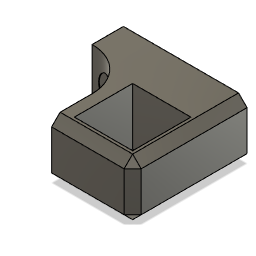
Hanger__Rod (Autodesk Fusion 360 design; units mm, degrees)
Autodesk Fusion 360 part; units mm, degrees
note: some values were not read from the file. Set by a fixed rule: which sketch regions a step uses.
sketch "Sketch1" plane through (0, 0, 0) normal (0, 1, 0) x (1, 0, 0)
  line L0 (0, 0) -> (20.5, 0)
  line L1 (20.5, 0) -> (20.5, -20.5)
  line L2 (20.5, -20.5) -> (0, -20.5)
  line L3 (0, -20.5) -> (0, 0)
  line L4 (0, 0) -> (-4, 0)
  line L5 (-4, 0) -> (-4, 4)
  line L6 (-4, 4) -> (0, 4)
  line L7 (0, 4) -> (0, 0)
  line L8 (-4, 4) -> (24.5, 4)
  line L9 (24.5, 4) -> (24.5, -24.5)
  line L10 (24.5, -24.5) -> (-4, -24.5)
  line L11 (-4, -24.5) -> (-4, 4)
  dimension "d1" = 20.5
  dimension "d2" = 20.5
  dimension "d3" = 4
  dimension "d4" = 4
  dimension "d5" = 28.5
  dimension "d6" = 28.5
  constraint horizontal L0
  constraint vertical L1
  constraint horizontal L2
  constraint vertical L3
  constraint coincident L0.start L3.end
  constraint horizontal L4
  constraint vertical L5
  constraint horizontal L6
  constraint vertical L7
  constraint horizontal L8
  constraint vertical L9
  constraint horizontal L10
  constraint vertical L11
  measures "d1" distance of L0.start L0.end
  measures "d2" distance of L0.start L2.end
  measures "d3" distance of L0.start L4.end
  measures "d4" distance of L0.start L6.end
  measures "d5" distance of L5.end L8.end
  measures "d6" distance of L5.end L10.end
extrude "Extrude1" add sketch "Sketch1" along normal blind 20
chamfer "Chamfer1" distance 3 angle 45 5 edges at (24.5, 20, 10.25) (10.25, 20, 24.5) (24.5, 10, 24.5) (24.5, 0, 10.25) (10.25, 0, 24.5)
sketch "Sketch2" plane through (0, 0, -4) normal (0, 0, -1) x (-1, 0, 0)
  line L0 (-24.5, 3) -> (-21.5, 0)
  line L1 (-21.5, 0) -> (4, 0)
  line L2 (4, 0) -> (4, 20)
  line L3 (4, 20) -> (-21.5, 20)
  line L4 (-21.5, 20) -> (-24.5, 17)
  line L5 (-24.5, 17) -> (-24.5, 3)
  line L6 (-24.5, 10) -> (-10.25, 10)
  line L7 (-7.6519, 5.5) -> (-5.0538, 10)
  line L8 (-5.0538, 10) -> (-7.6519, 14.5)
  line L9 (-7.6519, 14.5) -> (-12.8481, 14.5)
  line L10 (-12.8481, 14.5) -> (-15.4462, 10)
  line L11 (-15.4462, 10) -> (-12.8481, 5.5)
  line L12 (-12.8481, 5.5) -> (-7.6519, 5.5)
  point P0 (-10.25, 10)
  dimension "d10" = 14.25
  dimension "d11" = 4.5
  constraint midpoint L5 L6.start
  constraint perpendicular L2 L6
  constraint coincident P0 L6.end
  measures "d10" distance of L6.start P0
  measures "d11" distance of P0 L12
extrude "Extrude2" add sketch "Sketch2" along normal blind 4
sketch "Sketch3" plane through (0, 0, -8) normal (0, 0, -1) x (-1, 0, 0)
  line L0 (-7.6519, 5.5) -> (-12.8481, 5.5)
  line L1 (-15.4462, 10) -> (-12.8481, 14.5)
  line L2 (-12.8481, 14.5) -> (-7.6519, 14.5)
  line L3 (-7.6519, 14.5) -> (-5.0538, 10)
  line L4 (-5.0538, 10) -> (-7.6519, 5.5)
  line L5 (-24.5, 17) -> (-24.5, 3)
  line L6 (-24.5, 3) -> (-21.5, 0)
  line L7 (-21.5, 0) -> (4, 0)
  line L8 (4, 0) -> (4, 20)
  line L9 (4, 20) -> (-21.5, 20)
  line L10 (-21.5, 20) -> (-24.5, 17)
  line L11 (-7.6519, 14.5) -> (-5.0538, 14.5)
  line L12 (-5.0538, 14.5) -> (-5.0538, 10)
  line L13 (-15.4462, 10) -> (-15.4462, 14.5)
  line L14 (-15.4462, 14.5) -> (-12.8481, 14.5)
  constraint coincident L2.end L3.start
  constraint parallel L2 L11
  constraint coincident L3.end L4.start
  constraint perpendicular L11 L12
  constraint coincident L1.start L13.start
  constraint perpendicular L2 L13
  constraint coincident L1.end L2.start
  constraint perpendicular L13 L14
extrude "Extrude3" cut sketch "Sketch3" against normal blind 4 contours L1 L13 L14 | L3 L11 L12
sketch "Sketch4" plane through (0, 0, -8) normal (0, 0, -1) x (-1, 0, 0)
  line L0 (-15.4462, 14.5) -> (-5.0538, 14.5)
  line L1 (-5.0538, 14.5) -> (-5.0538, 10)
  line L2 (-5.0538, 10) -> (-7.6519, 5.5)
  line L3 (-7.6519, 5.5) -> (-12.8481, 5.5)
  line L4 (-12.8481, 5.5) -> (-15.4462, 10)
  line L5 (-15.4462, 10) -> (-15.4462, 14.5)
  line L6 (-24.5, 17) -> (-24.5, 3)
  line L7 (-24.5, 3) -> (-21.5, 0)
  line L8 (-21.5, 0) -> (4, 0)
  line L9 (4, 0) -> (4, 20)
  line L10 (4, 20) -> (-21.5, 20)
  line L11 (-21.5, 20) -> (-24.5, 17)
  line L12 (-10.25, 5.5) -> (-10.25, 10)
  circle A0 centre (-10.25, 10) radius 2
  line L13 (-5.0538, 14.5) -> (-15.4186, 14.5)
  line L14 (-15.4186, 14.5) -> (-15.4186, 5.5)
  line L15 (-15.4186, 5.5) -> (-5.0538, 5.5)
  line L16 (-5.0538, 5.5) -> (-5.0538, 14.5)
  line L17 (7, 22) -> (-27, 22)
  line L18 (-27, 22) -> (-27, -2)
  line L19 (-27, -2) -> (7, -2)
  line L20 (7, -2) -> (7, 22)
  dimension "d16" = 4
  constraint midpoint L3 L12.start
  constraint perpendicular L0 L12
  constraint coincident L12.end A0.centre
  constraint horizontal L13
  constraint vertical L14
  constraint horizontal L15
  constraint vertical L16
  constraint coincident L0.end L1.start
  constraint horizontal L17
  constraint vertical L18
  constraint horizontal L19
  constraint vertical L20
  measures "d16" diameter of A0
extrude "Extrude4" add sketch "Sketch4" along normal blind 5 contours L0 L1 L2 L3 L4 L13 L14 L15 L16 | L4 L14 L15 | L2 L15 L16 | L6 L7 L8 L9 L10 L11
extrude "Extrude5" add 1 faces at (0.0833, 10, -13) along direction (0, 0, -1) blind 1.75
sketch "Sketch5" plane through (-4, 0, 0) normal (-1, 0, 0) x (0, 0, 1)
  line L0 (21.5, 0) -> (24.5, 3)
  line L1 (24.5, 3) -> (24.5, 17)
  line L2 (24.5, 17) -> (21.5, 20)
  line L3 (21.5, 20) -> (-14.75, 20)
  line L4 (-14.75, 20) -> (-14.75, 0)
  line L5 (-14.75, 0) -> (21.5, 0)
  line L6 (-14.75, 20) -> (-4.75, 20)
  line L7 (-4.75, 20) -> (-4.75, 0)
  line L8 (-4.75, 0) -> (-14.75, 0)
  line L9 (-14.75, 0) -> (-14.75, 20)
  dimension "d21" = 10
  constraint horizontal L6
  constraint vertical L7
  constraint horizontal L8
  constraint vertical L9
  constraint coincident L3.end L4.start
  measures "d21" distance of L3.end L6.end
extrude "Extrude6" add sketch "Sketch5" along normal blind 15 contours L3 L4 L5 L6 L7 L8 L9
sketch "Sketch6" plane through (0, 0, -4.75) normal (0, 0, 1) x (1, 0, 0)
  line L0 (-4, 0) -> (-4, 20)
  line L1 (-4, 20) -> (-19, 20)
  line L2 (-19, 20) -> (-19, 0)
  line L3 (-19, 0) -> (-4, 0)
  line L4 (-19, 10) -> (-11.5, 10)
  circle A0 centre (-11.5, 10) radius 3.5
  dimension "d24" = 7.5
  dimension "d25" = 7
  constraint midpoint L2 L4.start
  constraint perpendicular L2 L4
  constraint coincident L4.end A0.centre
  measures "d24" distance of L4.start L4.end
  measures "d25" diameter of A0
extrude "Extrude7" cut sketch "Sketch6" against normal blind 10 contours A0
sketch "Sketch7" plane through (0, 0, 0) normal (0, -1, 0) x (1, 0, 0)
  line L0 (21.5, -14.75) -> (21.5, 21.5)
  line L1 (21.5, 21.5) -> (-4, 21.5)
  line L2 (-4, 21.5) -> (-4, -4.75)
  line L3 (-4, -4.75) -> (-19, -4.75)
  line L4 (-19, -4.75) -> (-19, -14.75)
  line L5 (-19, -14.75) -> (21.5, -14.75)
  line L6 (0, 20.5) -> (20.5, 20.5)
  line L7 (20.5, 20.5) -> (20.5, 0)
  line L8 (20.5, 0) -> (0, 0)
  line L9 (0, 0) -> (0, 20.5)
  line L10 (-19, -4.75) -> (-19, 10.25)
  circle A0 centre (-19, 10.25) radius 15
  dimension "d28" = 15
  constraint coincident L3.end L4.start
  constraint perpendicular L3 L10
  constraint coincident L10.end A0.centre
  constraint coincident L3.end A0
  measures "d28" distance of L3.end L10.end
extrude "Extrude8" add sketch "Sketch7" against normal blind 20 contours L2 L3 A0
sketch "Sketch8" plane through (0, 0, -14.75) normal (0, 0, -1) x (-1, 0, 0)
  circle A0 centre (11.5, 10) radius 3.5
  line L0 (-15.4462, 14.5) -> (-15.4186, 14.5)
  line L1 (-15.4186, 14.5) -> (-15.4186, 9.9523)
  line L2 (-15.4186, 9.9523) -> (-15.4462, 10)
  line L3 (-15.4462, 10) -> (-15.4462, 14.5)
  circle A1 centre (-10.25, 10) radius 2
  line L4 (-21.5, 20) -> (-24.5, 17)
  line L5 (-24.5, 17) -> (-24.5, 3)
  line L6 (-24.5, 3) -> (-21.5, 0)
  line L7 (-21.5, 0) -> (19, 0)
  line L8 (19, 0) -> (19, 20)
  line L9 (19, 20) -> (-21.5, 20)
  circle A2 centre (11.5, 10) radius 5
  dimension "d31" = 10
  constraint concentric A0 A2
  measures "d31" diameter of A2
extrude "Extrude9" cut sketch "Sketch8" along normal blind -10 and the other way blind 27 contours A2
extrude "Extrude10" cut 1 faces at (-11.9678, 9.7747, -4.75) along direction (0, 0, 1) blind 20
sketch "Sketch9" plane through (0, 0, -4.75) normal (0, 0, 1) x (1, 0, 0)
  circle A0 centre (-11.5, 10) radius 3.5
  circle A1 centre (-11.5, 10) radius 5
  circle A2 centre (-11.5, 10) radius 2
  dimension "d38" = 4
  constraint concentric A0 A2
  measures "d38" diameter of A2
extrude "Extrude11" add sketch "Sketch9" against normal blind 10 contours A0
sketch "Sketch10" plane through (0, 0, -4) normal (0, 0, -1) x (-1, 0, 0)
  line L0 (-7.6519, 5.5) -> (-5.0538, 10)
  line L1 (-5.0538, 10) -> (-5.0538, 14.5)
  line L2 (-5.0538, 14.5) -> (-15.4462, 14.5)
  line L3 (-15.4462, 14.5) -> (-15.4462, 10)
  line L4 (-15.4462, 10) -> (-12.8481, 5.5)
  line L5 (-12.8481, 5.5) -> (-7.6519, 5.5)
  line L6 (-10.25, 5.5) -> (-10.25, 10)
  circle A0 centre (-10.25, 10) radius 2
  dimension "d41" = 4
  constraint midpoint L5 L6.start
  constraint perpendicular L5 L6
  constraint coincident L6.end A0.centre
  measures "d41" diameter of A0
extrude "Extrude12" cut sketch "Sketch10" against normal blind 3.5 contours A0
extrude "Extrude13" add 1 faces at (9.7539, 10.3541, -0.5) along direction (0, 0, -1) blind 0.5
extrude "Extrude14" add 1 faces at (4.0064, 2.7128, -14.75) along direction (0, 0, -1) blind 1
sketch "Sketch11" plane through (0, 0, -4) normal (0, 0, -1) x (-1, 0, 0)
  circle A0 centre (-10.25, 10) radius 2
  line L0 (-7.6519, 5.5) -> (-5.0538, 10)
  line L1 (-5.0538, 10) -> (-5.0538, 14.5)
  line L2 (-5.0538, 14.5) -> (-15.4462, 14.5)
  line L3 (-15.4462, 14.5) -> (-15.4462, 10)
  line L4 (-15.4462, 10) -> (-12.8481, 5.5)
  line L5 (-12.8481, 5.5) -> (-7.6519, 5.5)
  line L6 (-8.5179, 7) -> (-6.7859, 10)
  line L7 (-6.7859, 10) -> (-8.5179, 13)
  line L8 (-8.5179, 13) -> (-11.9821, 13)
  line L9 (-11.9821, 13) -> (-13.7141, 10)
  line L10 (-13.7141, 10) -> (-11.9821, 7)
  line L11 (-11.9821, 7) -> (-8.5179, 7)
  line L12 (-6.7859, 10) -> (-13.7141, 10)
  line L13 (-13.7141, 10) -> (-13.7141, 13)
  line L14 (-13.7141, 13) -> (-6.7859, 13)
  line L15 (-6.7859, 13) -> (-6.7859, 10)
  point P0 (-10.25, 10)
  dimension "d48" = 3
  dimension "d49" = 3
  constraint coincident P0 A0.centre
  constraint horizontal L12
  constraint vertical L13
  constraint horizontal L14
  constraint vertical L15
  measures "d48" distance of P0 L11
  measures "d49" distance of L6.end L14.end
extrude "Extrude15" add sketch "Sketch11" along normal blind 5
extrude "Extrude16" add 1 faces at (13.16, 11.2893, -4) along direction (0, 0, -1) blind 1.5
extrude "Extrude17" add 1 faces at (15.4278, 11.4841, -9) along direction (0, 0, -1) blind 6.75
